Autodesk Fusion 360 part; units mm, degrees
(part 2 of 2)
  spline S12 degree 5 poles (8.4354, 4.1409) (8.4423, 4.1443) (8.4561, 4.1514) (8.4764, 4.1627) (8.5027, 4.179) (8.5346, 4.2013) (8.5657, 4.2248) (8.5964, 4.2491) (8.6268, 4.2738) (8.6571, 4.2989) (8.6872, 4.3243) (8.7171, 4.3501) (8.7466, 4.3765) (8.7757, 4.4035) (8.8044, 4.4311) (8.8328, 4.4593) (8.8608, 4.4879) (8.8886, 4.517) (8.9162, 4.5465) (8.9435, 4.5763) (8.9705, 4.6064) (8.9973, 4.6369) (9.0239, 4.6678) (9.0502, 4.699) (9.0762, 4.7307) (9.1019, 4.7627) (9.1274, 4.795) (9.1526, 4.8277) (9.1776, 4.8607) (9.2024, 4.894) (9.2269, 4.9276) (9.2511, 4.9615) (9.2752, 4.9957) (9.299, 5.0303) (9.3225, 5.0651) (9.3458, 5.1002) (9.3688, 5.1356) (9.3917, 5.1712) (9.4142, 5.2072) (9.4366, 5.2434) (9.4587, 5.2799) (9.4806, 5.3166) (9.5022, 5.3536) (9.5236, 5.3908) (9.5448, 5.4283) (9.5657, 5.4661) (9.5864, 5.5041) (9.6069, 5.5424) (9.6271, 5.5808) (9.6471, 5.6196) (9.6668, 5.6585) (9.6864, 5.6977) (9.7056, 5.7371) (9.7247, 5.7768) (9.7435, 5.8166) (9.7621, 5.8567) (9.7804, 5.897) (9.7986, 5.9376) (9.8164, 5.9783) (9.8341, 6.0192) (9.8515, 6.0604) (9.8686, 6.1017) (9.8856, 6.1433) (9.9023, 6.1851) (9.9187, 6.227) (9.935, 6.2692) (9.951, 6.3115) (9.9667, 6.3541) (9.9822, 6.3968) (9.9975, 6.4398) (10.0126, 6.4829) (10.0244, 6.5175) (10.0332, 6.5436) (10.039, 6.561) (10.0419, 6.5697) knots 0 0 0 0 0 0 0.01428571 0.02857143 0.04285714 0.05714286 0.07142857 0.08571429 0.1 0.11428571 0.12857143 0.14285714 0.15714286 0.17142857 0.18571429 0.2 0.21428571 0.22857143 0.24285714 0.25714286 0.27142857 0.28571429 0.3 0.31428571 0.32857143 0.34285714 0.35714286 0.37142857 0.38571429 0.4 0.41428571 0.42857143 0.44285714 0.45714286 0.47142857 0.48571429 0.5 0.51428571 0.52857143 0.54285714 0.55714286 0.57142857 0.58571429 0.6 0.61428571 0.62857143 0.64285714 0.65714286 0.67142857 0.68571429 0.7 0.71428571 0.72857143 0.74285714 0.75714286 0.77142857 0.78571429 0.8 0.81428571 0.82857143 0.84285714 0.85714286 0.87142857 0.88571429 0.9 0.91428571 0.92857143 0.94285714 0.95714286 0.97142857 0.98571429 1 1 1 1 1 1
  arc A26 (10.0419, 6.5697) -> (9.3513, 7.5202) centre (0, 0) ccw
  spline S13 degree 5 poles (9.3513, 7.5202) (9.3421, 7.5202) (9.3237, 7.52) (9.2962, 7.5198) (9.2596, 7.5192) (9.214, 7.5182) (9.1684, 7.5169) (9.123, 7.5154) (9.0777, 7.5136) (9.0324, 7.5114) (8.9873, 7.509) (8.9423, 7.5063) (8.8974, 7.5034) (8.8527, 7.5001) (8.808, 7.4965) (8.7635, 7.4927) (8.7191, 7.4886) (8.6749, 7.4842) (8.6307, 7.4795) (8.5867, 7.4745) (8.5429, 7.4692) (8.4991, 7.4636) (8.4555, 7.4577) (8.4121, 7.4516) (8.3688, 7.4451) (8.3256, 7.4384) (8.2826, 7.4313) (8.2398, 7.424) (8.1971, 7.4164) (8.1545, 7.4084) (8.1122, 7.4002) (8.07, 7.3916) (8.0279, 7.3828) (7.986, 7.3737) (7.9443, 7.3642) (7.9028, 7.3544) (7.8615, 7.3444) (7.8203, 7.334) (7.7793, 7.3233) (7.7386, 7.3123) (7.698, 7.301) (7.6576, 7.2894) (7.6174, 7.2774) (7.5775, 7.2652) (7.5377, 7.2526) (7.4982, 7.2396) (7.4588, 7.2264) (7.4197, 7.2128) (7.3809, 7.1989) (7.3422, 7.1847) (7.3038, 7.1701) (7.2657, 7.1551) (7.2279, 7.1398) (7.1903, 7.1241) (7.153, 7.108) (7.116, 7.0916) (7.0792, 7.0748) (7.0427, 7.0577) (7.0064, 7.0403) (6.9705, 7.0225) (6.9349, 7.0042) (6.8998, 6.9854) (6.8651, 6.9661) (6.8309, 6.9462) (6.7971, 6.9257) (6.7637, 6.905) (6.7305, 6.8839) (6.6975, 6.8626) (6.6649, 6.8409) (6.633, 6.8186) (6.602, 6.7952) (6.5783, 6.7752) (6.5613, 6.7594) (6.5503, 6.7485) (6.5449, 6.7429) knots -1 -1 -1 -1 -1 -1 -0.98571429 -0.97142857 -0.95714286 -0.94285714 -0.92857143 -0.91428571 -0.9 -0.88571429 -0.87142857 -0.85714286 -0.84285714 -0.82857143 -0.81428571 -0.8 -0.78571429 -0.77142857 -0.75714286 -0.74285714 -0.72857143 -0.71428571 -0.7 -0.68571429 -0.67142857 -0.65714286 -0.64285714 -0.62857143 -0.61428571 -0.6 -0.58571429 -0.57142857 -0.55714286 -0.54285714 -0.52857143 -0.51428571 -0.5 -0.48571429 -0.47142857 -0.45714286 -0.44285714 -0.42857143 -0.41428571 -0.4 -0.38571429 -0.37142857 -0.35714286 -0.34285714 -0.32857143 -0.31428571 -0.3 -0.28571429 -0.27142857 -0.25714286 -0.24285714 -0.22857143 -0.21428571 -0.2 -0.18571429 -0.17142857 -0.15714286 -0.14285714 -0.12857143 -0.11428571 -0.1 -0.08571429 -0.07142857 -0.05714286 -0.04285714 -0.02857143 -0.01428571 0 0 0 0 0 0
  line L13 (6.5449, 6.7429) -> (5.9123, 6.0924)
  arc A27 (4.5876, 5.9953) -> (5.9123, 6.0924) centre (5.1953, 6.7895) ccw
  arc A28 (4.5876, 5.9953) -> (4.2842, 6.2158) centre (0, 0) ccw
  arc A29 (3.9672, 7.5055) -> (4.2842, 6.2158) centre (4.8518, 7.0391) ccw
  line L14 (3.9672, 7.5055) -> (4.3904, 8.3082)
  spline S14 degree 5 poles (4.3904, 8.3082) (4.394, 8.3151) (4.401, 8.3289) (4.4108, 8.35) (4.4225, 8.3787) (4.4352, 8.4154) (4.4465, 8.4527) (4.4571, 8.4904) (4.4672, 8.5283) (4.4769, 8.5664) (4.4863, 8.6046) (4.4953, 8.6431) (4.5037, 8.6817) (4.5114, 8.7207) (4.5184, 8.7599) (4.5248, 8.7994) (4.5306, 8.8391) (4.536, 8.879) (4.541, 8.919) (4.5455, 8.9591) (4.5497, 8.9994) (4.5535, 9.0398) (4.5568, 9.0804) (4.5597, 9.1212) (4.5621, 9.162) (4.5641, 9.2031) (4.5657, 9.2442) (4.567, 9.2855) (4.5678, 9.3269) (4.5682, 9.3683) (4.5683, 9.4099) (4.568, 9.4516) (4.5673, 9.4934) (4.5663, 9.5353) (4.5649, 9.5773) (4.5631, 9.6194) (4.5609, 9.6616) (4.5584, 9.7039) (4.5556, 9.7462) (4.5524, 9.7887) (4.5488, 9.8312) (4.5449, 9.8738) (4.5407, 9.9164) (4.5361, 9.9591) (4.5312, 10.0019) (4.5259, 10.0448) (4.5203, 10.0877) (4.5144, 10.1306) (4.5081, 10.1737) (4.5016, 10.2167) (4.4946, 10.2599) (4.4874, 10.303) (4.4798, 10.3463) (4.4719, 10.3895) (4.4637, 10.4329) (4.4552, 10.4762) (4.4464, 10.5196) (4.4372, 10.563) (4.4277, 10.6065) (4.4179, 10.65) (4.4078, 10.6935) (4.3974, 10.7371) (4.3867, 10.7806) (4.3756, 10.8242) (4.3643, 10.8679) (4.3526, 10.9115) (4.3407, 10.9552) (4.3284, 10.9989) (4.3158, 11.0426) (4.303, 11.0863) (4.2898, 11.13) (4.279, 11.165) (4.2708, 11.1912) (4.2653, 11.2087) (4.2625, 11.2175) knots 0 0 0 0 0 0 0.01428571 0.02857143 0.04285714 0.05714286 0.07142857 0.08571429 0.1 0.11428571 0.12857143 0.14285714 0.15714286 0.17142857 0.18571429 0.2 0.21428571 0.22857143 0.24285714 0.25714286 0.27142857 0.28571429 0.3 0.31428571 0.32857143 0.34285714 0.35714286 0.37142857 0.38571429 0.4 0.41428571 0.42857143 0.44285714 0.45714286 0.47142857 0.48571429 0.5 0.51428571 0.52857143 0.54285714 0.55714286 0.57142857 0.58571429 0.6 0.61428571 0.62857143 0.64285714 0.65714286 0.67142857 0.68571429 0.7 0.71428571 0.72857143 0.74285714 0.75714286 0.77142857 0.78571429 0.8 0.81428571 0.82857143 0.84285714 0.85714286 0.87142857 0.88571429 0.9 0.91428571 0.92857143 0.94285714 0.95714286 0.97142857 0.98571429 1 1 1 1 1 1
  arc A30 (4.2625, 11.2175) -> (3.145, 11.5805) centre (0, 0) ccw
  spline S15 degree 5 poles (3.145, 11.5805) (3.1376, 11.5751) (3.1229, 11.5642) (3.1008, 11.5478) (3.0715, 11.5258) (3.0352, 11.4982) (2.9991, 11.4704) (2.9632, 11.4424) (2.9276, 11.4143) (2.8923, 11.386) (2.8572, 11.3575) (2.8224, 11.3289) (2.7878, 11.3001) (2.7535, 11.2712) (2.7195, 11.2421) (2.6857, 11.2128) (2.6522, 11.1834) (2.619, 11.1538) (2.5861, 11.124) (2.5534, 11.0941) (2.521, 11.0641) (2.4889, 11.0339) (2.4571, 11.0035) (2.4256, 10.973) (2.3944, 10.9423) (2.3634, 10.9115) (2.3328, 10.8805) (2.3024, 10.8494) (2.2724, 10.8181) (2.2426, 10.7867) (2.2132, 10.7551) (2.184, 10.7234) (2.1552, 10.6915) (2.1267, 10.6595) (2.0985, 10.6273) (2.0707, 10.595) (2.0431, 10.5626) (2.0159, 10.53) (1.9891, 10.4973) (1.9625, 10.4644) (1.9364, 10.4314) (1.9105, 10.3983) (1.885, 10.365) (1.8599, 10.3316) (1.8352, 10.298) (1.8108, 10.2643) (1.7868, 10.2305) (1.7631, 10.1965) (1.7398, 10.1624) (1.7169, 10.1282) (1.6945, 10.0938) (1.6724, 10.0593) (1.6508, 10.0246) (1.6296, 9.9899) (1.6089, 9.9549) (1.5886, 9.9199) (1.5687, 9.8847) (1.5492, 9.8494) (1.5301, 9.814) (1.5115, 9.7785) (1.4935, 9.7428) (1.4761, 9.7069) (1.4594, 9.6709) (1.4435, 9.6347) (1.4282, 9.5983) (1.4133, 9.5618) (1.3988, 9.5253) (1.3847, 9.4887) (1.371, 9.452) (1.3583, 9.4151) (1.347, 9.378) (1.3396, 9.3479) (1.3351, 9.3251) (1.3326, 9.3098) (1.3315, 9.3021) knots -1 -1 -1 -1 -1 -1 -0.98571429 -0.97142857 -0.95714286 -0.94285714 -0.92857143 -0.91428571 -0.9 -0.88571429 -0.87142857 -0.85714286 -0.84285714 -0.82857143 -0.81428571 -0.8 -0.78571429 -0.77142857 -0.75714286 -0.74285714 -0.72857143 -0.71428571 -0.7 -0.68571429 -0.67142857 -0.65714286 -0.64285714 -0.62857143 -0.61428571 -0.6 -0.58571429 -0.57142857 -0.55714286 -0.54285714 -0.52857143 -0.51428571 -0.5 -0.48571429 -0.47142857 -0.45714286 -0.44285714 -0.42857143 -0.41428571 -0.4 -0.38571429 -0.37142857 -0.35714286 -0.34285714 -0.32857143 -0.31428571 -0.3 -0.28571429 -0.27142857 -0.25714286 -0.24285714 -0.22857143 -0.21428571 -0.2 -0.18571429 -0.17142857 -0.15714286 -0.14285714 -0.12857143 -0.11428571 -0.1 -0.08571429 -0.07142857 -0.05714286 -0.04285714 -0.02857143 -0.01428571 0 0 0 0 0 0
  line L15 (1.3315, 9.3021) -> (1.2021, 8.404)
  arc A31 (0.1875, 7.5469) -> (1.2021, 8.404) centre (0.2123, 8.5466) ccw
  arc A32 (0.1875, 7.5469) -> (-0.1875, 7.5469) centre (0, 0) ccw
  arc A33 (-1.2021, 8.404) -> (-0.1875, 7.5469) centre (-0.2123, 8.5466) ccw
  line L16 (-1.2021, 8.404) -> (-1.3315, 9.3021)
  spline S16 degree 5 poles (-1.3315, 9.3021) (-1.3326, 9.3098) (-1.3351, 9.3251) (-1.3396, 9.3479) (-1.347, 9.378) (-1.3583, 9.4151) (-1.371, 9.452) (-1.3847, 9.4887) (-1.3988, 9.5253) (-1.4133, 9.5618) (-1.4282, 9.5983) (-1.4435, 9.6347) (-1.4594, 9.6709) (-1.4761, 9.7069) (-1.4935, 9.7428) (-1.5115, 9.7785) (-1.5301, 9.814) (-1.5492, 9.8494) (-1.5687, 9.8847) (-1.5886, 9.9199) (-1.6089, 9.9549) (-1.6296, 9.9899) (-1.6508, 10.0246) (-1.6724, 10.0593) (-1.6945, 10.0938) (-1.7169, 10.1282) (-1.7398, 10.1624) (-1.7631, 10.1965) (-1.7868, 10.2305) (-1.8108, 10.2643) (-1.8352, 10.298) (-1.8599, 10.3316) (-1.885, 10.365) (-1.9105, 10.3983) (-1.9364, 10.4314) (-1.9625, 10.4644) (-1.9891, 10.4973) (-2.0159, 10.53) (-2.0431, 10.5626) (-2.0707, 10.595) (-2.0985, 10.6273) (-2.1267, 10.6595) (-2.1552, 10.6915) (-2.184, 10.7234) (-2.2132, 10.7551) (-2.2426, 10.7867) (-2.2724, 10.8181) (-2.3024, 10.8494) (-2.3328, 10.8805) (-2.3634, 10.9115) (-2.3944, 10.9423) (-2.4256, 10.973) (-2.4571, 11.0035) (-2.4889, 11.0339) (-2.521, 11.0641) (-2.5534, 11.0941) (-2.5861, 11.124) (-2.619, 11.1538) (-2.6522, 11.1834) (-2.6857, 11.2128) (-2.7195, 11.2421) (-2.7535, 11.2712) (-2.7878, 11.3001) (-2.8224, 11.3289) (-2.8572, 11.3575) (-2.8923, 11.386) (-2.9276, 11.4143) (-2.9632, 11.4424) (-2.9991, 11.4704) (-3.0352, 11.4982) (-3.0715, 11.5258) (-3.1008, 11.5478) (-3.1229, 11.5642) (-3.1376, 11.5751) (-3.145, 11.5805) knots 0 0 0 0 0 0 0.01428571 0.02857143 0.04285714 0.05714286 0.07142857 0.08571429 0.1 0.11428571 0.12857143 0.14285714 0.15714286 0.17142857 0.18571429 0.2 0.21428571 0.22857143 0.24285714 0.25714286 0.27142857 0.28571429 0.3 0.31428571 0.32857143 0.34285714 0.35714286 0.37142857 0.38571429 0.4 0.41428571 0.42857143 0.44285714 0.45714286 0.47142857 0.48571429 0.5 0.51428571 0.52857143 0.54285714 0.55714286 0.57142857 0.58571429 0.6 0.61428571 0.62857143 0.64285714 0.65714286 0.67142857 0.68571429 0.7 0.71428571 0.72857143 0.74285714 0.75714286 0.77142857 0.78571429 0.8 0.81428571 0.82857143 0.84285714 0.85714286 0.87142857 0.88571429 0.9 0.91428571 0.92857143 0.94285714 0.95714286 0.97142857 0.98571429 1 1 1 1 1 1
  arc A34 (-3.145, 11.5805) -> (-4.2625, 11.2175) centre (0, 0) ccw
  spline S17 degree 5 poles (-4.2625, 11.2175) (-4.2653, 11.2087) (-4.2708, 11.1912) (-4.279, 11.165) (-4.2898, 11.13) (-4.303, 11.0863) (-4.3158, 11.0426) (-4.3284, 10.9989) (-4.3407, 10.9552) (-4.3526, 10.9115) (-4.3643, 10.8679) (-4.3756, 10.8242) (-4.3867, 10.7806) (-4.3974, 10.7371) (-4.4078, 10.6935) (-4.4179, 10.65) (-4.4277, 10.6065) (-4.4372, 10.563) (-4.4464, 10.5196) (-4.4552, 10.4762) (-4.4637, 10.4329) (-4.4719, 10.3895) (-4.4798, 10.3463) (-4.4874, 10.303) (-4.4946, 10.2599) (-4.5016, 10.2167) (-4.5081, 10.1737) (-4.5144, 10.1306) (-4.5203, 10.0877) (-4.5259, 10.0448) (-4.5312, 10.0019) (-4.5361, 9.9591) (-4.5407, 9.9164) (-4.5449, 9.8738) (-4.5488, 9.8312) (-4.5524, 9.7887) (-4.5556, 9.7462) (-4.5584, 9.7039) (-4.5609, 9.6616) (-4.5631, 9.6194) (-4.5649, 9.5773) (-4.5663, 9.5353) (-4.5673, 9.4934) (-4.568, 9.4516) (-4.5683, 9.4099) (-4.5682, 9.3683) (-4.5678, 9.3269) (-4.567, 9.2855) (-4.5657, 9.2442) (-4.5641, 9.2031) (-4.5621, 9.162) (-4.5597, 9.1212) (-4.5568, 9.0804) (-4.5535, 9.0398) (-4.5497, 8.9994) (-4.5455, 8.9591) (-4.541, 8.919) (-4.536, 8.879) (-4.5306, 8.8391) (-4.5248, 8.7994) (-4.5184, 8.7599) (-4.5114, 8.7207) (-4.5037, 8.6817) (-4.4953, 8.6431) (-4.4863, 8.6046) (-4.4769, 8.5664) (-4.4672, 8.5283) (-4.4571, 8.4904) (-4.4465, 8.4527) (-4.4352, 8.4154) (-4.4225, 8.3787) (-4.4108, 8.35) (-4.401, 8.3289) (-4.394, 8.3151) (-4.3904, 8.3082) knots -1 -1 -1 -1 -1 -1 -0.98571429 -0.97142857 -0.95714286 -0.94285714 -0.92857143 -0.91428571 -0.9 -0.88571429 -0.87142857 -0.85714286 -0.84285714 -0.82857143 -0.81428571 -0.8 -0.78571429 -0.77142857 -0.75714286 -0.74285714 -0.72857143 -0.71428571 -0.7 -0.68571429 -0.67142857 -0.65714286 -0.64285714 -0.62857143 -0.61428571 -0.6 -0.58571429 -0.57142857 -0.55714286 -0.54285714 -0.52857143 -0.51428571 -0.5 -0.48571429 -0.47142857 -0.45714286 -0.44285714 -0.42857143 -0.41428571 -0.4 -0.38571429 -0.37142857 -0.35714286 -0.34285714 -0.32857143 -0.31428571 -0.3 -0.28571429 -0.27142857 -0.25714286 -0.24285714 -0.22857143 -0.21428571 -0.2 -0.18571429 -0.17142857 -0.15714286 -0.14285714 -0.12857143 -0.11428571 -0.1 -0.08571429 -0.07142857 -0.05714286 -0.04285714 -0.02857143 -0.01428571 0 0 0 0 0 0
  line L17 (-4.3904, 8.3082) -> (-3.9672, 7.5055)
  arc A35 (-4.2842, 6.2158) -> (-3.9672, 7.5055) centre (-4.8518, 7.0391) ccw
  arc A36 (-4.2842, 6.2158) -> (-4.5876, 5.9953) centre (0, 0) ccw
  arc A37 (-5.9123, 6.0924) -> (-4.5876, 5.9953) centre (-5.1953, 6.7895) ccw
  line L18 (-5.9123, 6.0924) -> (-6.5449, 6.7429)
  spline S18 degree 5 poles (-6.5449, 6.7429) (-6.5503, 6.7485) (-6.5613, 6.7594) (-6.5783, 6.7752) (-6.602, 6.7952) (-6.633, 6.8186) (-6.6649, 6.8409) (-6.6975, 6.8626) (-6.7305, 6.8839) (-6.7637, 6.905) (-6.7971, 6.9257) (-6.8309, 6.9462) (-6.8651, 6.9661) (-6.8998, 6.9854) (-6.9349, 7.0042) (-6.9705, 7.0225) (-7.0064, 7.0403) (-7.0427, 7.0577) (-7.0792, 7.0748) (-7.116, 7.0916) (-7.153, 7.108) (-7.1903, 7.1241) (-7.2279, 7.1398) (-7.2657, 7.1551) (-7.3038, 7.1701) (-7.3422, 7.1847) (-7.3809, 7.1989) (-7.4197, 7.2128) (-7.4588, 7.2264) (-7.4982, 7.2396) (-7.5377, 7.2526) (-7.5775, 7.2652) (-7.6174, 7.2774) (-7.6576, 7.2894) (-7.698, 7.301) (-7.7386, 7.3123) (-7.7793, 7.3233) (-7.8203, 7.334) (-7.8615, 7.3444) (-7.9028, 7.3544) (-7.9443, 7.3642) (-7.986, 7.3737) (-8.0279, 7.3828) (-8.07, 7.3916) (-8.1122, 7.4002) (-8.1545, 7.4084) (-8.1971, 7.4164) (-8.2398, 7.424) (-8.2826, 7.4313) (-8.3256, 7.4384) (-8.3688, 7.4451) (-8.4121, 7.4516) (-8.4555, 7.4577) (-8.4991, 7.4636) (-8.5429, 7.4692) (-8.5867, 7.4745) (-8.6307, 7.4795) (-8.6749, 7.4842) (-8.7191, 7.4886) (-8.7635, 7.4927) (-8.808, 7.4965) (-8.8527, 7.5001) (-8.8974, 7.5034) (-8.9423, 7.5063) (-8.9873, 7.509) (-9.0324, 7.5114) (-9.0777, 7.5136) (-9.123, 7.5154) (-9.1684, 7.5169) (-9.214, 7.5182) (-9.2596, 7.5192) (-9.2962, 7.5198) (-9.3237, 7.52) (-9.3421, 7.5202) (-9.3513, 7.5202) knots 0 0 0 0 0 0 0.01428571 0.02857143 0.04285714 0.05714286 0.07142857 0.08571429 0.1 0.11428571 0.12857143 0.14285714 0.15714286 0.17142857 0.18571429 0.2 0.21428571 0.22857143 0.24285714 0.25714286 0.27142857 0.28571429 0.3 0.31428571 0.32857143 0.34285714 0.35714286 0.37142857 0.38571429 0.4 0.41428571 0.42857143 0.44285714 0.45714286 0.47142857 0.48571429 0.5 0.51428571 0.52857143 0.54285714 0.55714286 0.57142857 0.58571429 0.6 0.61428571 0.62857143 0.64285714 0.65714286 0.67142857 0.68571429 0.7 0.71428571 0.72857143 0.74285714 0.75714286 0.77142857 0.78571429 0.8 0.81428571 0.82857143 0.84285714 0.85714286 0.87142857 0.88571429 0.9 0.91428571 0.92857143 0.94285714 0.95714286 0.97142857 0.98571429 1 1 1 1 1 1
  arc A38 (-9.3513, 7.5202) -> (-10.0419, 6.5697) centre (0, 0) ccw
  spline S19 degree 5 poles (-10.0419, 6.5697) (-10.039, 6.561) (-10.0332, 6.5436) (-10.0244, 6.5175) (-10.0126, 6.4829) (-9.9975, 6.4398) (-9.9822, 6.3968) (-9.9667, 6.3541) (-9.951, 6.3115) (-9.935, 6.2692) (-9.9187, 6.227) (-9.9023, 6.1851) (-9.8856, 6.1433) (-9.8686, 6.1017) (-9.8515, 6.0604) (-9.8341, 6.0192) (-9.8164, 5.9783) (-9.7986, 5.9376) (-9.7804, 5.897) (-9.7621, 5.8567) (-9.7435, 5.8166) (-9.7247, 5.7768) (-9.7056, 5.7371) (-9.6864, 5.6977) (-9.6668, 5.6585) (-9.6471, 5.6196) (-9.6271, 5.5808) (-9.6069, 5.5424) (-9.5864, 5.5041) (-9.5657, 5.4661) (-9.5448, 5.4283) (-9.5236, 5.3908) (-9.5022, 5.3536) (-9.4806, 5.3166) (-9.4587, 5.2799) (-9.4366, 5.2434) (-9.4142, 5.2072) (-9.3917, 5.1712) (-9.3688, 5.1356) (-9.3458, 5.1002) (-9.3225, 5.0651) (-9.299, 5.0303) (-9.2752, 4.9957) (-9.2511, 4.9615) (-9.2269, 4.9276) (-9.2024, 4.894) (-9.1776, 4.8607) (-9.1526, 4.8277) (-9.1274, 4.795) (-9.1019, 4.7627) (-9.0762, 4.7307) (-9.0502, 4.699) (-9.0239, 4.6678) (-8.9973, 4.6369) (-8.9705, 4.6064) (-8.9435, 4.5763) (-8.9162, 4.5465) (-8.8886, 4.517) (-8.8608, 4.4879) (-8.8328, 4.4593) (-8.8044, 4.4311) (-8.7757, 4.4035) (-8.7466, 4.3765) (-8.7171, 4.3501) (-8.6872, 4.3243) (-8.6571, 4.2989) (-8.6268, 4.2738) (-8.5964, 4.2491) (-8.5657, 4.2248) (-8.5346, 4.2013) (-8.5027, 4.179) (-8.4764, 4.1627) (-8.4561, 4.1514) (-8.4423, 4.1443) (-8.4354, 4.1409) knots -1 -1 -1 -1 -1 -1 -0.98571429 -0.97142857 -0.95714286 -0.94285714 -0.92857143 -0.91428571 -0.9 -0.88571429 -0.87142857 -0.85714286 -0.84285714 -0.82857143 -0.81428571 -0.8 -0.78571429 -0.77142857 -0.75714286 -0.74285714 -0.72857143 -0.71428571 -0.7 -0.68571429 -0.67142857 -0.65714286 -0.64285714 -0.62857143 -0.61428571 -0.6 -0.58571429 -0.57142857 -0.55714286 -0.54285714 -0.52857143 -0.51428571 -0.5 -0.48571429 -0.47142857 -0.45714286 -0.44285714 -0.42857143 -0.41428571 -0.4 -0.38571429 -0.37142857 -0.35714286 -0.34285714 -0.32857143 -0.31428571 -0.3 -0.28571429 -0.27142857 -0.25714286 -0.24285714 -0.22857143 -0.21428571 -0.2 -0.18571429 -0.17142857 -0.15714286 -0.14285714 -0.12857143 -0.11428571 -0.1 -0.08571429 -0.07142857 -0.05714286 -0.04285714 -0.02857143 -0.01428571 0 0 0 0 0 0
  line L19 (-8.4354, 4.1409) -> (-7.6212, 3.7403)
  arc A39 (-7.1196, 2.5104) -> (-7.6212, 3.7403) centre (-8.0626, 2.843) ccw
  circle A40 centre (0, 0) radius 17.5
  dimension "d9" = 35
  constraint concentric A0 A40
  measures "d9" diameter of A40
extrude "Extrude3" add sketch "Sketch1 (2)" along normal blind 7 contours A0 A1 L0 S0 A2 S1 L1 A3 A4 A5 L2 S2 A6 S3 L3 A7 A8 A9 L4 S4 A10 S5 L5 A11 A12 A13 L6 S6 A14 S7 L7 A15 A16 A17 L8 S8 A18 S9 L9 A19 A20 A21 L10 S10 A22 S11 L11 A23 A24 A25 L12 S12 A26 S13 L13 A27 A28 A29 L14 S14 A30 S15 L15 A31 A32 A33 L16 S16 A34 S17 L17 A35 A36 A37 L18 S18 A38 S19 L19 A39 | A40 in component "Spur Gear (10 teeth)"
sketch "Sketch2 (2)" plane through (0, 0, 38) normal (0, 0, 1) x (-1, 0, 0)
  line L0 (-3.5, -6.0622) -> (3.5, -6.0622)
  line L1 (3.5, -6.0622) -> (7, 0)
  line L2 (7, 0) -> (3.5, 6.0622)
  line L3 (3.5, 6.0622) -> (-3.5, 6.0622)
  line L4 (-3.5, 6.0622) -> (-7, 0)
  line L5 (-7, 0) -> (-3.5, -6.0622)
  circle A0 centre (0, 0) radius 5.75
extrude "Extrude4" cut sketch "Sketch2 (2)" against normal blind 31 contours L0 L1 L2 L3 L4 L5 | A0 in component "Spur Gear (10 teeth)"
component "Spur Gear (10 teeth)" placed x (1, 0, 0) y (0, 1, 0) z (0, 0, 1) at (0, 0, 0)

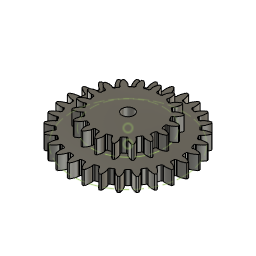
design "front axle gear"
description: Spur Gear; Module: 2.0; Num Teeth: 28; Pressure Angle: 20.0; Backlash: 1.00 mm
description: Spur Gear; Module: 2.0; Num Teeth: 18; Pressure Angle: 20.0; Backlash: 1.00 mm
Autodesk Fusion 360 part; units mm, degrees
sketch "Sketch1" plane through (0, 0, 0) normal (0, 0, 1) x (1, 0, 0) in component "Spur Gear (28 teeth)"
  circle A0 centre (0, 0) radius 25.5492
  circle A1 centre (0, 0) radius 3
extrude "Extrude1" add sketch "Sketch1" along normal blind 7 makes body 1 in component "Spur Gear (28 teeth)"
sketch "Sketch2" plane through (0, 0, 0) normal (0, 0, 1) x (1, 0, 0) in component "Spur Gear (28 teeth)"
  spline S0 degree 5 poles (26.2607, -1.6322) (26.2715, -1.6329) (26.2931, -1.634) (26.3254, -1.6348) (26.3686, -1.6345) (26.4225, -1.632) (26.4765, -1.6281) (26.5306, -1.6233) (26.5846, -1.618) (26.6386, -1.6123) (26.6927, -1.6063) (26.7467, -1.5999) (26.8008, -1.5928) (26.8548, -1.5851) (26.9089, -1.5767) (26.9629, -1.5676) (27.0169, -1.5579) (27.0709, -1.5478) (27.1249, -1.5372) (27.1789, -1.5263) (27.2329, -1.515) (27.2868, -1.5033) (27.3407, -1.4912) (27.3946, -1.4786) (27.4485, -1.4656) (27.5024, -1.4522) (27.5562, -1.4384) (27.61, -1.4242) (27.6638, -1.4097) (27.7176, -1.3948) (27.7714, -1.3795) (27.8251, -1.3639) (27.8788, -1.348) (27.9324, -1.3317) (27.9861, -1.315) (28.0397, -1.298) (28.0933, -1.2807) (28.1468, -1.2631) (28.2003, -1.2451) (28.2538, -1.2269) (28.3073, -1.2083) (28.3607, -1.1894) (28.414, -1.1702) (28.4674, -1.1507) (28.5207, -1.1308) (28.574, -1.1107) (28.6272, -1.0903) (28.6804, -1.0696) (28.7336, -1.0486) (28.7867, -1.0273) (28.8398, -1.0058) (28.8928, -0.9839) (28.9458, -0.9618) (28.9988, -0.9394) (29.0517, -0.9167) (29.1046, -0.8937) (29.1574, -0.8705) (29.2102, -0.847) (29.2629, -0.8232) (29.3156, -0.7992) (29.3683, -0.7749) (29.4209, -0.7503) (29.4735, -0.7255) (29.526, -0.7004) (29.5785, -0.6751) (29.6309, -0.6495) (29.6832, -0.6236) (29.7356, -0.5975) (29.7878, -0.5711) (29.8401, -0.5445) (29.8922, -0.5177) (29.9339, -0.496) (29.9652, -0.4796) (29.986, -0.4686) (29.9964, -0.4631) knots 0 0 0 0 0 0 0.01428571 0.02857143 0.04285714 0.05714286 0.07142857 0.08571429 0.1 0.11428571 0.12857143 0.14285714 0.15714286 0.17142857 0.18571429 0.2 0.21428571 0.22857143 0.24285714 0.25714286 0.27142857 0.28571429 0.3 0.31428571 0.32857143 0.34285714 0.35714286 0.37142857 0.38571429 0.4 0.41428571 0.42857143 0.44285714 0.45714286 0.47142857 0.48571429 0.5 0.51428571 0.52857143 0.54285714 0.55714286 0.57142857 0.58571429 0.6 0.61428571 0.62857143 0.64285714 0.65714286 0.67142857 0.68571429 0.7 0.71428571 0.72857143 0.74285714 0.75714286 0.77142857 0.78571429 0.8 0.81428571 0.82857143 0.84285714 0.85714286 0.87142857 0.88571429 0.9 0.91428571 0.92857143 0.94285714 0.95714286 0.97142857 0.98571429 1 1 1 1 1 1
  spline S1 degree 5 poles (26.2607, 1.6322) (26.2715, 1.6329) (26.2931, 1.634) (26.3254, 1.6348) (26.3686, 1.6345) (26.4225, 1.632) (26.4765, 1.6281) (26.5306, 1.6233) (26.5846, 1.618) (26.6386, 1.6123) (26.6927, 1.6063) (26.7467, 1.5999) (26.8008, 1.5928) (26.8548, 1.5851) (26.9089, 1.5767) (26.9629, 1.5676) (27.0169, 1.5579) (27.0709, 1.5478) (27.1249, 1.5372) (27.1789, 1.5263) (27.2329, 1.515) (27.2868, 1.5033) (27.3407, 1.4912) (27.3946, 1.4786) (27.4485, 1.4656) (27.5024, 1.4522) (27.5562, 1.4384) (27.61, 1.4242) (27.6638, 1.4097) (27.7176, 1.3948) (27.7714, 1.3795) (27.8251, 1.3639) (27.8788, 1.348) (27.9324, 1.3317) (27.9861, 1.315) (28.0397, 1.298) (28.0933, 1.2807) (28.1468, 1.2631) (28.2003, 1.2451) (28.2538, 1.2269) (28.3073, 1.2083) (28.3607, 1.1894) (28.414, 1.1702) (28.4674, 1.1507) (28.5207, 1.1308) (28.574, 1.1107) (28.6272, 1.0903) (28.6804, 1.0696) (28.7336, 1.0486) (28.7867, 1.0273) (28.8398, 1.0058) (28.8928, 0.9839) (28.9458, 0.9618) (28.9988, 0.9394) (29.0517, 0.9167) (29.1046, 0.8937) (29.1574, 0.8705) (29.2102, 0.847) (29.2629, 0.8232) (29.3156, 0.7992) (29.3683, 0.7749) (29.4209, 0.7503) (29.4735, 0.7255) (29.526, 0.7004) (29.5785, 0.6751) (29.6309, 0.6495) (29.6832, 0.6236) (29.7356, 0.5975) (29.7878, 0.5711) (29.8401, 0.5445) (29.8922, 0.5177) (29.9339, 0.496) (29.9652, 0.4796) (29.986, 0.4686) (29.9964, 0.4631) knots 0 0 0 0 0 0 0.01428571 0.02857143 0.04285714 0.05714286 0.07142857 0.08571429 0.1 0.11428571 0.12857143 0.14285714 0.15714286 0.17142857 0.18571429 0.2 0.21428571 0.22857143 0.24285714 0.25714286 0.27142857 0.28571429 0.3 0.31428571 0.32857143 0.34285714 0.35714286 0.37142857 0.38571429 0.4 0.41428571 0.42857143 0.44285714 0.45714286 0.47142857 0.48571429 0.5 0.51428571 0.52857143 0.54285714 0.55714286 0.57142857 0.58571429 0.6 0.61428571 0.62857143 0.64285714 0.65714286 0.67142857 0.68571429 0.7 0.71428571 0.72857143 0.74285714 0.75714286 0.77142857 0.78571429 0.8 0.81428571 0.82857143 0.84285714 0.85714286 0.87142857 0.88571429 0.9 0.91428571 0.92857143 0.94285714 0.95714286 0.97142857 0.98571429 1 1 1 1 1 1
  arc A0 (29.9964, -0.4631) -> (29.9964, 0.4631) centre (0, 0) ccw
  line L0 (25.49, -1.585) -> (26.2607, -1.6322)
  line L1 (25.49, 1.585) -> (26.2607, 1.6322)
  line L2 (25.49, -1.585) -> (25.49, 1.585)
  point P0 (26.5252, -1.6236)
  point P1 (26.791, -1.594)
  point P2 (27.0574, -1.5502)
  point P3 (27.3244, -1.4948)
  point P4 (27.5918, -1.429)
  point P5 (27.8594, -1.3537)
  point P6 (28.1271, -1.2696)
  point P7 (28.3948, -1.1771)
  point P8 (28.6624, -1.0766)
  point P9 (28.9299, -0.9684)
  point P10 (29.1971, -0.8528)
  point P11 (29.464, -0.7299)
  point P12 (29.7305, -0.6)
  point P13 (26.5252, 1.6236)
  point P14 (26.791, 1.594)
  point P15 (27.0574, 1.5502)
  point P16 (27.3244, 1.4948)
  point P17 (27.5918, 1.429)
  point P18 (27.8594, 1.3537)
  point P19 (28.1271, 1.2696)
  point P20 (28.3948, 1.1771)
  point P21 (28.6624, 1.0766)
  point P22 (28.9299, 0.9684)
  point P23 (29.1971, 0.8528)
  point P24 (29.464, 0.7299)
  point P25 (29.7305, 0.6)
extrude "Extrude2" add sketch "Sketch2" along normal blind 7 bodies 1 in component "Spur Gear (28 teeth)"
fillet "Fillet1" radius 0.5 2 edges at (25.5, -1.5856, 3.5) (25.5, 1.5856, 3.5) on bodies 1 in component "Spur Gear (28 teeth)"
pattern_circular "C-Pattern1" count 28 over 360 about axis through (0, 0, 0) along (0, 0, 1) of "Extrude2", "Fillet1" in component "Spur Gear (28 teeth)"
sketch "Sketch3" plane through (0, 0, 0) normal (0, 0, 1) x (1, 0, 0) in component "Spur Gear (28 teeth)"
  circle A0 centre (0, 0) radius 28 construction
sketch "Sketch1 (2)" plane through (0, 0, 0) normal (0, 0, 1) x (1, 0, 0) in component "Spur Gear (18 teeth)"
  circle A0 centre (0, 0) radius 15.5492
  circle A1 centre (0, 0) radius 3
extrude "Extrude1'" add sketch "Sketch1 (2)" along normal blind 7 separate body makes body 2 in component "Spur Gear (18 teeth)"
sketch "Sketch2 (2)" plane through (0, 0, 0) normal (0, 0, 1) x (1, 0, 0) in component "Spur Gear (18 teeth)"
  spline S0 degree 5 poles (16.8486, -1.4913) (16.8576, -1.4921) (16.8758, -1.4934) (16.9029, -1.4947) (16.9392, -1.495) (16.9846, -1.4934) (17.0301, -1.4904) (17.0756, -1.4866) (17.1212, -1.4823) (17.1668, -1.4776) (17.2123, -1.4726) (17.2579, -1.4672) (17.3035, -1.4612) (17.3491, -1.4545) (17.3947, -1.4471) (17.4403, -1.4391) (17.486, -1.4305) (17.5316, -1.4215) (17.5772, -1.4121) (17.6227, -1.4023) (17.6683, -1.3922) (17.7139, -1.3816) (17.7594, -1.3706) (17.805, -1.3592) (17.8505, -1.3474) (17.896, -1.3352) (17.9415, -1.3226) (17.987, -1.3096) (18.0324, -1.2962) (18.0778, -1.2825) (18.1232, -1.2685) (18.1686, -1.2541) (18.214, -1.2394) (18.2593, -1.2243) (18.3046, -1.2089) (18.3498, -1.1931) (18.3951, -1.177) (18.4403, -1.1606) (18.4855, -1.1439) (18.5306, -1.1268) (18.5757, -1.1095) (18.6208, -1.0918) (18.6658, -1.0739) (18.7108, -1.0556) (18.7558, -1.037) (18.8007, -1.0181) (18.8456, -0.999) (18.8904, -0.9795) (18.9352, -0.9598) (18.98, -0.9397) (19.0247, -0.9194) (19.0694, -0.8988) (19.114, -0.8779) (19.1586, -0.8567) (19.2031, -0.8353) (19.2476, -0.8135) (19.292, -0.7916) (19.3364, -0.7693) (19.3808, -0.7468) (19.4251, -0.724) (19.4693, -0.7009) (19.5135, -0.6776) (19.5576, -0.654) (19.6017, -0.6301) (19.6457, -0.606) (19.6897, -0.5816) (19.7336, -0.557) (19.7775, -0.5321) (19.8213, -0.507) (19.865, -0.4816) (19.9087, -0.4559) (19.9436, -0.4352) (19.9698, -0.4196) (19.9872, -0.4091) (19.9959, -0.4039) knots 0 0 0 0 0 0 0.01428571 0.02857143 0.04285714 0.05714286 0.07142857 0.08571429 0.1 0.11428571 0.12857143 0.14285714 0.15714286 0.17142857 0.18571429 0.2 0.21428571 0.22857143 0.24285714 0.25714286 0.27142857 0.28571429 0.3 0.31428571 0.32857143 0.34285714 0.35714286 0.37142857 0.38571429 0.4 0.41428571 0.42857143 0.44285714 0.45714286 0.47142857 0.48571429 0.5 0.51428571 0.52857143 0.54285714 0.55714286 0.57142857 0.58571429 0.6 0.61428571 0.62857143 0.64285714 0.65714286 0.67142857 0.68571429 0.7 0.71428571 0.72857143 0.74285714 0.75714286 0.77142857 0.78571429 0.8 0.81428571 0.82857143 0.84285714 0.85714286 0.87142857 0.88571429 0.9 0.91428571 0.92857143 0.94285714 0.95714286 0.97142857 0.98571429 1 1 1 1 1 1
  spline S1 degree 5 poles (16.8486, 1.4913) (16.8576, 1.4921) (16.8758, 1.4934) (16.9029, 1.4947) (16.9392, 1.495) (16.9846, 1.4934) (17.0301, 1.4904) (17.0756, 1.4866) (17.1212, 1.4823) (17.1668, 1.4776) (17.2123, 1.4726) (17.2579, 1.4672) (17.3035, 1.4612) (17.3491, 1.4545) (17.3947, 1.4471) (17.4403, 1.4391) (17.486, 1.4305) (17.5316, 1.4215) (17.5772, 1.4121) (17.6227, 1.4023) (17.6683, 1.3922) (17.7139, 1.3816) (17.7594, 1.3706) (17.805, 1.3592) (17.8505, 1.3474) (17.896, 1.3352) (17.9415, 1.3226) (17.987, 1.3096) (18.0324, 1.2962) (18.0778, 1.2825) (18.1232, 1.2685) (18.1686, 1.2541) (18.214, 1.2394) (18.2593, 1.2243) (18.3046, 1.2089) (18.3498, 1.1931) (18.3951, 1.177) (18.4403, 1.1606) (18.4855, 1.1439) (18.5306, 1.1268) (18.5757, 1.1095) (18.6208, 1.0918) (18.6658, 1.0739) (18.7108, 1.0556) (18.7558, 1.037) (18.8007, 1.0181) (18.8456, 0.999) (18.8904, 0.9795) (18.9352, 0.9598) (18.98, 0.9397) (19.0247, 0.9194) (19.0694, 0.8988) (19.114, 0.8779) (19.1586, 0.8567) (19.2031, 0.8353) (19.2476, 0.8135) (19.292, 0.7916) (19.3364, 0.7693) (19.3808, 0.7468) (19.4251, 0.724) (19.4693, 0.7009) (19.5135, 0.6776) (19.5576, 0.654) (19.6017, 0.6301) (19.6457, 0.606) (19.6897, 0.5816) (19.7336, 0.557) (19.7775, 0.5321) (19.8213, 0.507) (19.865, 0.4816) (19.9087, 0.4559) (19.9436, 0.4352) (19.9698, 0.4196) (19.9872, 0.4091) (19.9959, 0.4039) knots 0 0 0 0 0 0 0.01428571 0.02857143 0.04285714 0.05714286 0.07142857 0.08571429 0.1 0.11428571 0.12857143 0.14285714 0.15714286 0.17142857 0.18571429 0.2 0.21428571 0.22857143 0.24285714 0.25714286 0.27142857 0.28571429 0.3 0.31428571 0.32857143 0.34285714 0.35714286 0.37142857 0.38571429 0.4 0.41428571 0.42857143 0.44285714 0.45714286 0.47142857 0.48571429 0.5 0.51428571 0.52857143 0.54285714 0.55714286 0.57142857 0.58571429 0.6 0.61428571 0.62857143 0.64285714 0.65714286 0.67142857 0.68571429 0.7 0.71428571 0.72857143 0.74285714 0.75714286 0.77142857 0.78571429 0.8 0.81428571 0.82857143 0.84285714 0.85714286 0.87142857 0.88571429 0.9 0.91428571 0.92857143 0.94285714 0.95714286 0.97142857 0.98571429 1 1 1 1 1 1
  arc A0 (19.9959, -0.4039) -> (19.9959, 0.4039) centre (0, 0) ccw
  line L0 (15.4787, -1.3709) -> (16.8486, -1.4913)
  line L1 (15.4787, 1.3709) -> (16.8486, 1.4913)
  line L2 (15.4787, -1.3709) -> (15.4787, 1.3709)
  point P0 (17.0702, -1.4869)
  point P1 (17.2935, -1.4624)
  point P2 (17.5179, -1.4242)
  point P3 (17.7429, -1.3746)
  point P4 (17.9684, -1.3148)
  point P5 (18.1942, -1.2457)
  point P6 (18.4203, -1.1678)
  point P7 (18.6463, -1.0816)
  point P8 (18.8722, -0.9874)
  point P9 (19.0979, -0.8854)
  point P10 (19.3232, -0.7759)
  point P11 (19.5481, -0.659)
  point P12 (19.7724, -0.535)
  point P13 (17.0702, 1.4869)
  point P14 (17.2935, 1.4624)
  point P15 (17.5179, 1.4242)
  point P16 (17.7429, 1.3746)
  point P17 (17.9684, 1.3148)
  point P18 (18.1942, 1.2457)
  point P19 (18.4203, 1.1678)
  point P20 (18.6463, 1.0816)
  point P21 (18.8722, 0.9874)
  point P22 (19.0979, 0.8854)
  point P23 (19.3232, 0.7759)
  point P24 (19.5481, 0.659)
  point P25 (19.7724, 0.535)
extrude "Extrude2'" add sketch "Sketch2 (2)" along normal blind 7 bodies 2 in component "Spur Gear (18 teeth)"
fillet "Fillet1'" radius 0.5 2 edges at (15.4886, -1.3718, 3.5) (15.4886, 1.3718, 3.5) on bodies 2 in component "Spur Gear (18 teeth)"
pattern_circular "C-Pattern1'" count 18 over 360 about axis through (0, 0, 0) along (0, 0, 1) of "Extrude2'", "Fillet1'" in component "Spur Gear (18 teeth)"
sketch "Sketch3 (2)" plane through (0, 0, 0) normal (0, 0, 1) x (1, 0, 0) in component "Spur Gear (18 teeth)"
  circle A0 centre (0, 0) radius 18 construction
combine "Combine1" operation add target body 2 tool bodies 1 body 1 seen with x (1, 0, 0) y (0, 1, 0) z (0, 0, 1) at (0, 0, -7) in component "Spur Gear (18 teeth)"
component "Spur Gear (28 teeth)" placed x (1, 0, 0) y (0, 1, 0) z (0, 0, 1) at (0, 0, 0)
component "Spur Gear (18 teeth)" placed x (1, 0, 0) y (0, 1, 0) z (0, 0, 1) at (0, 0, 7)
